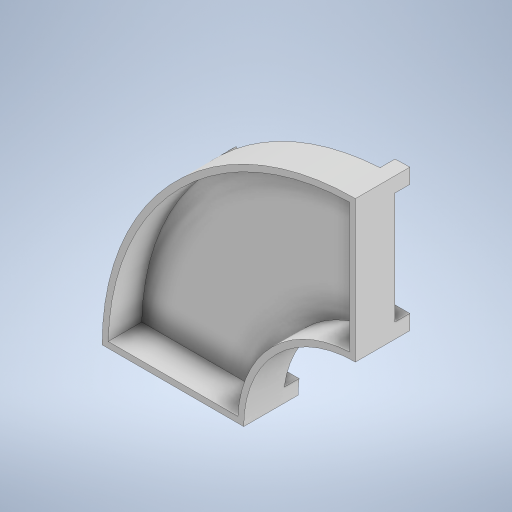
# Autodesk Inventor part: Bandeja Radial
Saved by Autodesk Inventor 2023 (Build 270158000, 158)
## iProperties
Created: 2023-03-08
Part Number: Bandeja Radial
Material: Genérico
Document SubType Name: Modeling
Designer: Inteli
Density: 1 g/cm^3
Appearance: Padrão
Author: Inteli
Autodesk Inventor part; units mm, degrees
ref_plane "YZ Plane" through (0, 0, 0) normal (1, 0, 0) x (0, 1, 0)
ref_plane "XZ Plane" through (0, 0, 0) normal (0, 1, 0) x (-1, 0, 0)
ref_plane "XY Plane" through (0, 0, 0) normal (0, 0, 1) x (1, 0, 0)
sketch "Esboço1" plane through (0, 0, 0) normal (0, 0, 1) x (1, 0, 0)
  arc A0 (0, 340) -> (-340, 0) centre (0, 0) ccw
  arc A1 (0, 150) -> (-150, 0) centre (0, 0) ccw
  line L0 (0, 0) -> (170, 0) construction
  line L1 (0, 0) -> (155, 0) construction
  line L2 (0, 0) -> (155, 0) construction
  line L3 (0, 340) -> (0, 150)
  line L4 (-150, 0) -> (-340, 0)
  arc A2 (-8, 157.7973) -> (-157.7973, 8) centre (0, 0) ccw
  line L5 (-8, 157.7973) -> (-8, 331.9036)
  arc A3 (-8, 331.9036) -> (-331.9036, 8) centre (0, 0) ccw
  line L6 (-331.9036, 8) -> (-157.7973, 8)
  dimension "d16" = 680
  dimension "d17" = 300
  dimension "d18" = 8
  constraints: 14 end point, 8 point on circle, 4 centre point, 3 horizontal, 2 coincident, 2 perpendicular, 1 vertical, 3 other
  measures "d16" diameter of A0
  measures "d17" diameter of A1
  measures "d18" radial gap between concentric circles of A1 A2
extrude "Parede" add sketch "Esboço1" along normal blind 45
extrude "Fundo" add sketch "Esboço1" against normal blind 8 contours L3 A1 L4 A0 | A2 L6 A3 L5
sketch "Esboço3" plane through (0, 0, -8) normal (0, 0, -1) x (-1, 0, 0)
  line L0 (150, 0) -> (340, 0) projected
  line L1 (150, 0) -> (170, 0)
  line L2 (170, 0) -> (170, 20)
  line L3 (170, 20) -> (148.6607, 20)
  arc A0 (150, 0) -> (0, 150) centre (0, 0) ccw projected
  arc A1 (150, 0) -> (148.6607, 20) centre (0, 0) ccw
  line L4 (0, 150) -> (0, 170)
  line L5 (0, 340) -> (0, 150) projected
  line L6 (0, 170) -> (20, 170)
  line L7 (20, 170) -> (20, 148.6607)
  arc A2 (20, 148.6607) -> (0, 150) centre (0, 0) ccw
  line L8 (0, 340) -> (0, 320)
  line L9 (0, 320) -> (20, 320)
  arc A3 (340, 0) -> (0, 340) centre (0, 0) ccw projected
  line L10 (20, 320) -> (20, 339.4113)
  arc A4 (20, 339.4113) -> (0, 340) centre (0, 0) ccw
  line L11 (340, 0) -> (320, 0)
  line L12 (320, 0) -> (320, 20)
  line L13 (320, 20) -> (339.4113, 20)
  arc A5 (340, 0) -> (339.4113, 20) centre (0, 0) ccw
  line L14 (247.3834, 233.2412) -> (233.3452, 219.2031)
  line L15 (233.2412, 247.3834) -> (219.2031, 233.3452)
  arc A6 (233.3452, 219.2031) -> (219.2031, 233.3452) centre (0.1105, 0.1105) ccw
  arc A7 (247.3834, 233.2412) -> (233.2412, 247.3834) centre (0, 0) ccw
  dimension "d23" = 20
  dimension "d24" = 20
  dimension "d25" = 20
  dimension "d26" = 20
  dimension "d27" = 20
  dimension "d28" = 20
  dimension "d29" = 20
  dimension "d30" = 20
  dimension "d34" = 320
  constraints: 28 end point, 19 point on circle, 7 perpendicular, 6 centre point, 6 concentric, 4 point on line, 1 vertical
  measures "d23" distance of L0.start L1.end
  measures "d24" distance of L1.end L2.end
  measures "d25" distance of L4.start L4.end
  measures "d26" distance of L4.end L6.end
  measures "d27" distance of L5.start L8.end
  measures "d28" distance of L8.end L9.end
  measures "d29" distance of L0.end L11.end
  measures "d30" distance of L11.end L12.end
  measures "d34" radius of A6
extrude "Extrusão6" add sketch "Esboço3" along normal blind 20 contours A0 L3 L2 L0 | L12 L13 A3 L0 | A0 L4 L6 L7 | L14 A6 L15 A3 | L5 A3 L10 L9
